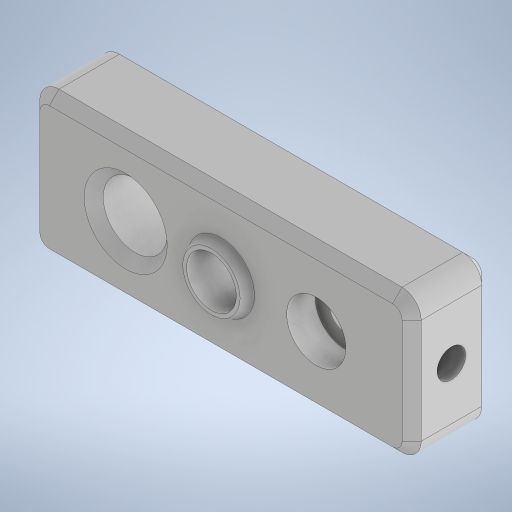
# Autodesk Inventor part: Z Idle belt
Saved by Autodesk Inventor 2023.1 (Build 271208000, 208)
## iProperties
Created: 2022-10-30
Part Number: Z Idle belt
Material: Generic
Document SubType Name: Modeling
Designer: nicol
Density: 1 g/cm^3
Appearance: Default
Author: nicol
Autodesk Inventor part; units mm, degrees
ref_plane "YZ Plane" through (0, 0, 0) normal (1, 0, 0) x (0, 1, 0)
ref_plane "XZ Plane" through (0, 0, 0) normal (0, 1, 0) x (-1, 0, 0)
ref_plane "XY Plane" through (0, 0, 0) normal (0, 0, 1) x (1, 0, 0)
sketch "Sketch1" plane through (0, 0, 0) normal (0, 0, 1) x (1, 0, 0)
  line L0 (0, 0) -> (40, 0)
  line L1 (40, 0) -> (40, 8.35)
  line L2 (40, 8.35) -> (0, 8.35)
  line L3 (0, 8.35) -> (0, 0)
  dimension "d0" = 40
  dimension "d1" = 8.35
  constraints: 8 end point, 2 parallel, 1 horizontal, 1 perpendicular
  measures "d0" distance of L0.start L0.end
  measures "d1" distance of L2.end L0.start
extrude "Extrusion1" add sketch "Sketch1" along normal blind 15
sketch "Sketch2" plane through (0, 8.35, 0) normal (0, 1, 0) x (1, 0, 0)
  line L0 (40, 0) -> (0, 0) projected
  line L1 (0, 0) -> (0, -15) projected
  line L2 (40, -15) -> (0, -15) projected
  line L3 (40, 0) -> (40, -15) projected
  line L4 (20, -2.7657) -> (24.1, -5.1329)
  line L5 (24.1, -5.1329) -> (24.1, -9.8671)
  line L6 (24.1, -9.8671) -> (20, -12.2343)
  line L7 (20, -12.2343) -> (15.9, -9.8671)
  line L8 (15.9, -9.8671) -> (15.9, -5.1329)
  line L9 (15.9, -5.1329) -> (20, -2.7657)
  point P0 (0, 0)
  point P1 (20, -7.5)
  point P2 (0, -7.5)
  point P3 (20, -15)
  dimension "d4" = 8.2
  constraints: 12 end point, 2 midpoint, 1 horizontal alignment, 1 vertical, 1 vertical alignment, 13 other
  measures "d4" distance between parallel lines of L4 L7
extrude "Extrusion2" cut sketch "Sketch2" against normal blind 5 contours L4 L5 L6 L7 L8 L9
hole "Hole1" at (20, 8.35, 7.5) direction (0, -1, 0) diameter 5.2 end through all
sketch "Sketch3" plane through (0, 0, 0) normal (0, -1, 0) x (1, 0, 0)
  circle A0 centre (20, 7.5) radius 2.6 projected
  line L0 (0, 0) -> (40, 0) projected
  line L1 (40, 0) -> (40, 15) projected
  line L2 (0, 15) -> (40, 15) projected
  line L3 (0, 0) -> (0, 15) projected
  circle A1 centre (20, 7.5) radius 3
  dimension "d14" = 6
  constraints: 1 centre point, 1 coincident
  measures "d14" diameter of A1
extrude "Extrusion3" add sketch "Sketch3" along normal blind 1 contours A1
chamfer "Chamfer3" distance 0.5 distance2 1 1 edges at (17, 0, 7.5) measured on face at (16.5, 0, 7.5)
sketch "Sketch4" plane through (0, 0, 0) normal (0, -1, 0) x (1, 0, 0)
  line L0 (0, 0) -> (40, 0) projected
  line L1 (40, 0) -> (40, 15) projected
  line L2 (0, 15) -> (40, 15) projected
  line L3 (0, 0) -> (0, 15) projected
  point P0 (10, 7.5)
  point P1 (30, 7.5)
  point P2 (0, 7.5)
  dimension "d20" = 10
  dimension "d21" = 10
  constraints: 2 horizontal alignment, 1 midpoint
  measures "d20" distance from line of L3 point (10, 7.5)
  measures "d21" distance from line of L1 point (30, 7.5)
hole "Hole2" at (10, 0, 7.5) direction (0, 1, 0) diameter 3.2 end through all counterbore diameter 6.2 counterbore depth 3
sketch "Sketch7" plane through (0, 3.35, 0) normal (0, 1, 0) x (1, 0, 0)
  circle A0 centre (20, -7.5) radius 2.6 projected
  line L0 (15.9, -9.8671) -> (15.9, -5.1329) projected
  line L1 (20, -12.2343) -> (15.9, -9.8671) projected
  line L2 (24.1, -9.8671) -> (20, -12.2343) projected
  line L3 (24.1, -5.1329) -> (24.1, -9.8671) projected
  line L4 (20, -2.7657) -> (24.1, -5.1329) projected
  line L5 (15.9, -5.1329) -> (20, -2.7657) projected
  line L6 (17.4, -4.2668) -> (17.4, -10.7332)
  line L7 (22.6, -4.2668) -> (22.6, -10.7332)
  circle A1 centre (20, -7.5) radius 2.6 projected
  point P0 (0, 0)
  point P1 (22.6, -7.5)
  point P2 (17.4, -7.5)
  constraints: 4 end point, 4 point on line, 2 tangent, 2 vertical
extrude "Extrusion4" cut sketch "Sketch7" against normal blind 0.2 contours L7 L2 L1 L6 A0 | A0 L6 L5 L4 L7
sketch "Sketch8" plane through (0, 3.15, 0) normal (0, 1, 0) x (1, 0, 0)
  line L0 (20, -2.7657) -> (22.6, -4.2668) projected
  line L1 (17.4, -4.2668) -> (20, -2.7657) projected
  line L2 (17.4, -7.5) -> (17.4, -4.2668) projected
  arc A0 (22.6, -7.5) -> (17.4, -7.5) centre (20, -7.5) ccw projected
  line L3 (22.6, -4.2668) -> (22.6, -7.5) projected
  arc A1 (17.4, -7.5) -> (22.6, -7.5) centre (20, -7.5) ccw projected
  line L4 (17.4, -10.7332) -> (17.4, -7.5) projected
  line L5 (20, -12.2343) -> (17.4, -10.7332) projected
  line L6 (22.6, -10.7332) -> (20, -12.2343) projected
  line L7 (22.6, -7.5) -> (22.6, -10.7332) projected
  line L8 (17.4, -10.1) -> (22.6, -10.1)
  line L9 (17.4, -4.9) -> (22.6, -4.9)
  arc A2 (22.6, -7.5) -> (17.4, -7.5) centre (20, -7.5) ccw projected
  point P0 (0, 0)
  point P1 (20, -4.9)
  point P2 (20, -10.1)
  constraints: 4 end point, 4 point on line, 2 horizontal, 2 tangent
extrude "Extrusion5" cut sketch "Sketch8" against normal blind 0.2 contours L3 A0 L9 | L9 A0 L2 | L7 L8 A1 | A1 L8 L4
hole "Hole3" at (30, 0, 7.5) direction (0, 1, 0) diameter 6.7 end through all
sketch "Sketch9" plane through (0, 0, 0) normal (-1, 0, 0) x (0, 0, 1)
  circle A0 centre (7.5, 4.175) radius 1.5
  line L0 (5.9, 8.35) -> (9.1, 8.35) projected
  line L1 (9.1, 8.35) -> (9.1, 0)
  line L2 (10.85, 0) -> (4.15, 0) projected
  line L3 (15, 8.35) -> (15, 0) projected
  point P0 (0, 0)
  point P1 (5.9, 0)
  point P2 (9.1, 4.175)
  point P3 (7.5, 8.35)
  dimension "d45" = 3
  constraints: 2 end point, 2 midpoint, 1 centre point, 1 horizontal alignment, 1 perpendicular, 1 vertical alignment
  measures "d45" diameter of A0
extrude "Extrusion6" cut sketch "Sketch9" against normal blind 5
fillet "Fillet1" radius 2 4 edges at (40, 4.175, 0) (40, 4.175, 15) (0, 4.175, 0) (0, 4.175, 15)
chamfer "Chamfer2" distance 1 angle 45 16 edges at (20, 8.35, 0) (0.5858, 8.35, 0.5858) (0, 8.35, 7.5) (0.5858, 8.35, 14.4142) (20, 8.35, 15) (39.4142, 8.35, 14.4142) (40, 8.35, 7.5) (39.4142, 8.35, 0.5858) (20, 0, 0) (39.4142, 0, 0.5858) (40, 0, 7.5) (39.4142, 0, 14.4142) (20, 0, 15) (0.5858, 0, 14.4142) (0, 0, 7.5) (0.5858, 0, 0.5858)
chamfer "Chamfer4" distance 1 angle 45 2 edges at (30, 0, 10.85) (30, 8.35, 10.85)
body "Solid1"
